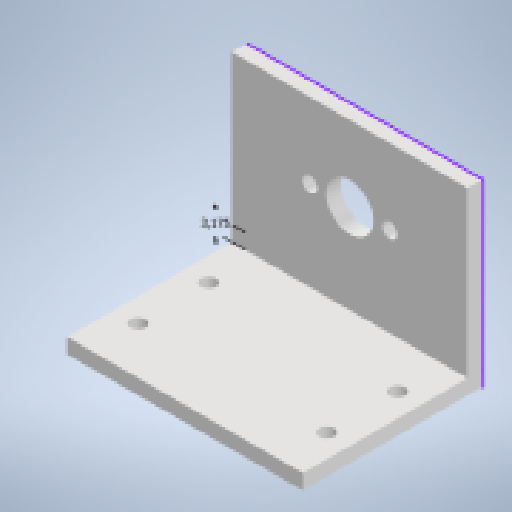
# Autodesk Inventor part: Suportepara o motor em cantorneira
Saved by Autodesk Inventor 2023 (Build 270158000, 158)
## iProperties
Created: 2022-10-11
Part Number: Suportepara o motor em cantorneira
Material: Generic
Document SubType Name: Modeling
Designer: klebe
Density: 1 g/cm^3
Appearance: Default
Description: Suporte em aço astm A36 - 1.1/2 x 1/8
Author: klebe
Autodesk Inventor part; units mm, degrees
ref_plane "YZ Plane" through (0, 0, 0) normal (1, 0, 0) x (0, 1, 0)
ref_plane "XZ Plane" through (0, 0, 0) normal (0, 1, 0) x (-1, 0, 0)
ref_plane "XY Plane" through (0, 0, 0) normal (0, 0, 1) x (1, 0, 0)
sketch "Sketch1" plane through (0, 0, 0) normal (0, 0, 1) x (1, 0, 0)
  line L0 (25, 16.8) -> (25, -19.8)
  line L1 (25, -19.8) -> (-25, -19.8)
  line L2 (-25, -19.8) -> (-25, 16.8)
  line L3 (-25, -19.8) -> (-25, -16.8)
  line L4 (-25, -19.8) -> (-25, 18.3)
  line L5 (-25, 18.3) -> (25, 18.3)
  line L6 (25, 18.3) -> (25, -19.8)
  line L7 (-25, -19.8) -> (-25, -16.625)
  line L8 (-25, -16.625) -> (25, -16.625)
  dimension "d94" = 3.175
  constraints: 18 end point, 3 point on line, 1 collinear, 1 horizontal, 1 parallel, 1 perpendicular, 1 vertical
  measures "d94" distance of L1.end L7.end
extrude "Extrusion3" add sketch "Sketch1" along normal blind 3.175
extrude "Extrusion4" add sketch "Sketch1" along normal blind 38.1 contours L0 L1 L2 L8
sketch "Sketch2" plane through (-25, -16.625, 3) normal (0, 1, 0) x (1, 0, 0)
  line L0 (50, -35.1) -> (0, -35.1) projected
  line L1 (0, 0) -> (50, 0) projected
  line L2 (0, 0) -> (0, -35.1) projected
  line L3 (50, 0) -> (50, -35.1) projected
  line L4 (50, -35.1) -> (45, -35.1)
  line L5 (0, -35.1) -> (0, -25.1)
  line L6 (0, 3) -> (0, -35.1) projected
  line L7 (45, -35.1) -> (45, -25.1)
  line L8 (45, -25.1) -> (5, -25.1)
  line L9 (5, -25.1) -> (5, -10.1)
  line L10 (5, -10.1) -> (45, -10.1)
  line L11 (45, -10.1) -> (45, -25.1)
  point P0 (40, -25.1)
  point P1 (40, -10)
  point P2 (10, -10)
  point P3 (10, -25.1)
  dimension "d83" = 5
  dimension "d84" = 10
  dimension "d85" = 40
  dimension "d86" = 15
  constraints: 14 end point, 2 parallel, 2 point on line, 1 horizontal, 1 perpendicular, 1 vertical
  measures "d83" distance of L0.start L4.end
  measures "d84" distance of L0.end L5.end
  measures "d85" distance of L9.end L10.end
  measures "d86" distance of L8.end L9.end
sketch "Sketch3" plane through (0, 0, 0) normal (0, 0, -1) x (-1, 0, 0)
  line L0 (25, 18.3) -> (25, -0.75)
  line L1 (-25, -16.8) -> (-25, 18.3) projected
  line L2 (25, 18.3) -> (25, 2.3)
  line L3 (25, 18.3) -> (25, -19.8) projected
  line L4 (0, 2.2) -> (0.1, 2.2)
  point P0 (0, -0.75)
  dimension "d89" = 4
  dimension "d67" = 19.05
  dimension "d68" = 25
  dimension "d95" = 16
  dimension "d98" = 0.1
  constraints: 6 end point, 1 point on line, 1 vertical
  measures "d67" distance of L0.start L0.end
  measures "d68" distance of L0.end point (0, -0.75)
  measures "d95" distance of L0.start L2.end
  measures "d98" distance of L4.start L4.end
hole "Hole4" at (0, 2.2, 0) direction (0, 0, 1) diameter 10 end through all
sketch "Sketch4" plane through (0, 0, 0) normal (0, 0, -1) x (-1, 0, 0)
  circle A0 centre (-8.5, -0.75) radius 1.2295 projected
  circle A1 centre (8.5, -0.75) radius 1.2295 projected
  line L0 (-25, 18.3) -> (25, 18.3) projected
  line L1 (25, 18.3) -> (25, 2.3)
  line L2 (25, 18.3) -> (25, -19.8) projected
  line L3 (8.5, 2.2) -> (-8.5, 2.1769)
  point P0 (0, 0)
  point P1 (8.5, 2.1769)
  dimension "d96" = 16
  constraints: 4 end point, 1 point on line
  measures "d96" distance of L0.end L1.end
hole "Hole5" at (8.5, 2.1769, 0) at (-8.5, 2.1769, 0) direction (0, 0, 1) diameter 3.18 end through all
hole "Hole6" at (20, -16.625, 28.1) at (20, -16.625, 13.1) at (-20, -16.625, 28.1) at (-20, -16.625, 13.1) direction (0, -1, 0) diameter 3.18 end through all
body "Solid2"
